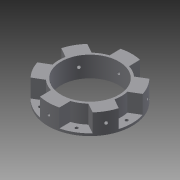
# Autodesk Inventor part: flangev4
Saved by Autodesk Inventor 2015 (Build 190159000, 159)
## iProperties
Created: 2016-04-16
Part Number: flangev4
Material: Generic
Document SubType Name: Modeling
Designer: ypatel4
Density: 1 g/cm^3
Appearance: Default
Author: ypatel4
Autodesk Inventor part; units mm, degrees
ref_plane "YZ Plane" through (0, 0, 0) normal (1, 0, 0) x (0, 1, 0)
ref_plane "XZ Plane" through (0, 0, 0) normal (0, 1, 0) x (-1, 0, 0)
sketch "Sketch1" plane through (0, 0, 0) normal (0, 1, 0) x (-1, 0, 0)
  circle A0 centre (0, 0) radius 61.087
  circle A1 centre (0, 0) radius 88.9
  dimension "d0" = 122.174
  dimension "d1" = 177.8
  constraints: 2 centre point, 2 coincident
  measures "d0" diameter of A0
  measures "d1" diameter of A1
extrude "Extrusion1" add sketch "Sketch1" along normal blind 5.08
sketch "Sketch2" plane through (0, 5.08, 0) normal (0, 1, 0) x (1, 0, 0)
  circle A0 centre (0, 0) radius 61.087 projected
  circle A1 centre (0, 0) radius 66.167
  dimension "d4" = 132.334
  dimension "d5" = 122.174
  constraints: 1 centre point, 1 coincident
  measures "d4" diameter of A1
  measures "d5" diameter of A0
extrude "Extrusion2" add sketch "Sketch2" along normal blind 38.354
sketch "Sketch3" plane through (0, 5.08, 0) normal (0, 1, 0) x (1, 0, 0)
  circle A0 centre (0, 0) radius 66.167 projected
  circle A1 centre (0, 0) radius 88.9 projected
  line L0 (66.167, 0) -> (88.9, 0) construction
  line L1 (66.167, 0) -> (77.5335, 0)
  circle A2 centre (77.5335, 0) radius 3.175
  point P0 (80.7085, 0)
  dimension "d10" = 6.35
  dimension "d8" = 22.733
  dimension "d9" = 11.3665
  dimension "d11" = 8.1915
  constraints: 4 end point, 3 horizontal alignment, 2 coincident, 1 horizontal, 1 midpoint, 1 point on line, 4 other
  measures "d8" distance of L0.start L0.end
  measures "d9" distance of L0.start L1.end
  measures "d11" distance of point (80.709, 0) point (88.9, 0)
hole "Hole1" at (77.5335, 5.08, 0) direction (0, -1, 0) diameter 6.35 end through all
pattern_circular "Circular Pattern1" count 6 over 360 about axis through (0, -10, 0) along (0, 1, 0) of "Hole1"
sketch "Sketch4" plane through (0, 5.08, 0) normal (0, 1, 0) x (1, 0, 0)
  circle A0 centre (0, 0) radius 66.167 projected
  line L0 (43.7225, 49.663) -> (63.9658, 61.7381)
  circle A1 centre (0, 0) radius 88.9 projected
  line L1 (64.5029, 14.7462) -> (84.7557, 26.827)
  arc A2 (64.5029, 14.7462) -> (41.6667, 51.4) centre (0, 0) ccw
  arc A3 (81.2449, 36.0899) -> (63.9658, 61.7381) centre (0, 0) ccw
  circle A4 centre (77.5335, 0) radius 3.175 projected
  circle A5 centre (38.7668, 67.146) radius 3.175 projected
  constraints: 10 point on circle, 4 end point, 2 centre point, 2 concentric, 1 parallel
extrude "Extrusion3" add sketch "Sketch4" along normal blind 38.354 contours A0 L0 A1 L1 picked at (52.8659, 51.2219)
ref_plane "Work Plane3" through (76.382, 43.434, -45.4862) normal (0.8591904, 0, -0.5116561) x (0, 1, 0)
sketch "Sketch6" plane through (76.382, 43.434, -45.4862) normal (0.8591904, 0, -0.5116561) x (0, 1, 0)
  line L0 (0, 61.087) -> (0, -61.087) projected
  line L1 (0, 0) -> (-21.717, 0)
  circle A0 centre (-21.717, 0) radius 3.175
  point P0 (-43.434, 0)
  dimension "d35" = 21.717
  dimension "d36" = 6.35
  constraints: 2 end point, 1 centre point, 1 coincident, 1 horizontal, 1 midpoint
  measures "d35" distance of L1.start L1.end
  measures "d36" diameter of A0
hole "Hole3" at (76.382, 21.717, -45.4862) direction (-0.8591904, 0, 0.5116561) diameter 6.35 depth 39.1795 tip angle 118
pattern_circular "Circular Pattern3" count 6 over 360 about axis through (0, -10, 0) along (0, 1, 0) of "Hole3", "Extrusion3"
body "Solid1"
